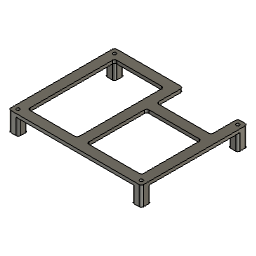
CCMDebugSupportv1 (Autodesk Fusion 360 design; units mm, degrees)
Autodesk Fusion 360 part; units mm, degrees
sketch "Sketch1" plane through (0, 0, 0) normal (0, 0, 1) x (1, 0, 0)
  line L0 (-60, 47.5) -> (60, 47.5)
  line L1 (60, 47.5) -> (60, -47.5)
  line L2 (60, -47.5) -> (-60, -47.5)
  line L3 (-60, -47.5) -> (-60, 47.5)
  line L4 (0, 66) -> (0, -78) construction
  line L5 (-80, 0) -> (100, 0) construction
  circle A0 centre (-57.5, 45) radius 1.5
  circle A1 centre (57.5, 45) radius 1.5
  circle A2 centre (-57.5, -45) radius 1.5
  circle A3 centre (57.5, -45) radius 1.5
  line L6 (62, -49.5) -> (-62, -49.5)
  line L7 (-62, -49.5) -> (-62, 49.5)
  line L8 (-62, 49.5) -> (62, 49.5)
  line L9 (62, 49.5) -> (62, -49.5)
  dimension "d1" = 120
  dimension "d2" = 95
  dimension "d3" = 3
  dimension "d4" = 2.5
  dimension "d5" = 2.5
  dimension "d8" = 115
  dimension "d9" = -90
  dimension "d12" = -2
  constraint horizontal L0
  constraint perpendicular L0 L1
  constraint parallel L0 L2
  constraint parallel L1 L3
  constraint perpendicular L2 L4
  constraint perpendicular L1 L5
  measures "d1" distance of L1.end L2.end
  measures "d2" distance of L0.end L1.end
  measures "d3" diameter of A0
  measures "d4" distance of L3 A0.centre
  measures "d5" distance of L0 A0.centre
extrude "Extrude1" add sketch "Sketch1" along normal blind 3 contours L0 L1 L2 L3
extrude "Extrude2" add sketch "Sketch1" along normal blind 3 contours L6 L7 L8 L9
sketch "Sketch2" plane through (0, 0, 3) normal (0, 0, 1) x (-1, 0, 0)
  line L0 (-62, -49.5) -> (62, -49.5)
  line L1 (62, -49.5) -> (62, 49.5)
  line L2 (62, 49.5) -> (-62, 49.5)
  line L3 (-62, 49.5) -> (-62, -49.5)
  circle A0 centre (57.5, -45) radius 1.5
  circle A1 centre (-57.5, -45) radius 1.5
  circle A2 centre (57.5, 45) radius 1.5
  circle A3 centre (-57.5, 45) radius 1.5
  line L4 (-2, -49.5) -> (-53, -49.5)
  line L5 (-53, -49.5) -> (-53, -24.5)
  line L6 (-53, -24.5) -> (-2, -24.5)
  line L7 (-2, -24.5) -> (-2, -49.5)
  dimension "d15" = 51
  dimension "d16" = 25
  dimension "d17" = 9
  constraint horizontal L4
  constraint vertical L5
  constraint horizontal L6
  constraint vertical L7
  constraint coincident L0 L4.start
  measures "d15" distance of L5.end L6.end
  measures "d16" distance of L4.start L6.end
  measures "d17" distance of L3 L5
extrude "Extrude3" cut sketch "Sketch2" against normal up to surface (3 mm away) contours L0 L4 L5 L6 L7
sketch "Sketch3" plane through (0, 0, 3) normal (0, 0, 1) x (-1, 0, 0)
  line L0 (-2, -24.5) -> (-2, -49.5)
  line L1 (-2, -49.5) -> (62, -49.5)
  line L2 (62, -49.5) -> (62, 49.5)
  line L3 (62, 49.5) -> (-62, 49.5)
  line L4 (-62, 49.5) -> (-62, -49.5)
  line L5 (-62, -49.5) -> (-53, -49.5)
  line L6 (-53, -49.5) -> (-53, -24.5)
  line L7 (-53, -24.5) -> (-2, -24.5)
  circle A0 centre (57.5, -45) radius 1.5
  circle A1 centre (-57.5, -45) radius 1.5
  circle A2 centre (57.5, 45) radius 1.5
  circle A3 centre (-57.5, 45) radius 1.5
  line L8 (53, -40.5) -> (7, -40.5)
  line L9 (7, -40.5) -> (7, 40.5)
  line L10 (7, 40.5) -> (53, 40.5)
  line L11 (53, 40.5) -> (53, -40.5)
  line L12 (-2, -15.5) -> (-53, -15.5)
  line L13 (-53, -15.5) -> (-53, 40.5)
  line L14 (-53, 40.5) -> (-2, 40.5)
  line L15 (-2, 40.5) -> (-2, -15.5)
  point P0 (57.5, -45)
  dimension "d20" = 4.5
  dimension "d21" = 4.5
  dimension "d22" = 4.5
  dimension "d23" = 4.5
  dimension "d24" = 9
  dimension "d25" = 4.5
  dimension "d27" = 9
  dimension "d28" = 9
  constraint horizontal L8
  constraint vertical L9
  constraint horizontal L10
  constraint vertical L11
  constraint horizontal L12
  constraint vertical L13
  constraint horizontal L14
  constraint vertical L15
  measures "d20" distance of P0 L8
  measures "d21" distance of L11 P0
  measures "d22" distance of A2.centre L10
  measures "d23" distance of A3.centre L13
  measures "d24" distance of L7 L12
  measures "d25" distance of A3.centre L14
  measures "d27" distance of L0 L9
  measures "d28" distance of L9 L15
extrude "Extrude4" cut sketch "Sketch3" against normal up to surface (3 mm away) contours L8 L9 L10 L11 | L12 L13 L14 L15
sketch "Sketch9" plane through (0, 0, 0) normal (0, 0, 1) x (1, 0, 0)
  line L0 (-62, -49.5) -> (-53, -49.5)
  line L1 (-53, -49.5) -> (-53, -40.5)
  line L2 (-53, -40.5) -> (-62, -40.5)
  line L3 (-62, -40.5) -> (-62, -49.5)
  line L4 (-62, -49.5) -> (-53, -40.5) construction
  line L5 (-53, -49.5) -> (-62, -40.5) construction
  line L6 (53, -49.5) -> (62, -49.5)
  line L7 (62, -49.5) -> (62, -40.5)
  line L8 (62, -40.5) -> (53, -40.5)
  line L9 (53, -40.5) -> (53, -49.5)
  line L10 (-62, 40.5) -> (-53, 40.5)
  line L11 (-53, 40.5) -> (-53, 49.5)
  line L12 (-53, 49.5) -> (-62, 49.5)
  line L13 (-62, 49.5) -> (-62, 40.5)
  line L14 (53, 40.5) -> (62, 40.5)
  line L15 (62, 40.5) -> (62, 49.5)
  line L16 (62, 49.5) -> (53, 49.5)
  line L17 (53, 49.5) -> (53, 40.5)
  point P0 (-57.5, -45)
  point P1 (-62, -49.5)
  point P2 (-57.5, -45)
  point P3 (57.5, -45)
  point P4 (-57.5, 45)
  point P5 (57.5, 45)
  dimension "d54" = 115
  dimension "d55" = 90
  constraint horizontal L0
  constraint perpendicular L0 L1
  constraint parallel L0 L2
  constraint parallel L1 L3
  constraint coincident L4 P2
  constraint coincident L5 P2
  constraint coincident L0.start L3.end
  constraint coincident P2 P0
extrude "Extrude10" add sketch "Sketch9" against normal blind 15
extrude "Extrude11" cut sketch "Sketch1" against normal up to surface (15 mm away) contours A0 | A1 | A2 | A3
fillet "Fillet1" radius 2 16 edges at (53, 49.5, -6) (2, 49.5, 1.5) (-53, 49.5, -7.5) (-62, 49.5, -6) (-62, -40.5, -7.5) (-53, -40.5, -7.5) (62, -40.5, -7.5) (53, -40.5, -7.5) (53, -49.5, -7.5) (-53, 40.5, -7.5) (53, 40.5, -7.5) (62, 40.5, -7.5) (-62, 40.5, -7.5) (-62, -49.5, -6) (62, -49.5, -6) (62, 49.5, -6)
fillet "Fillet2" radius 2 1 edges at (-53, -49.5, -7.5)
fillet "Fillet3" radius 2 10 edges at (53, 24.5, 1.5) (53, -40.5, 1.5) (53, 15.5, 1.5) (-7, 40.5, 1.5) (-7, -40.5, 1.5) (-53, -40.5, 1.5) (2, 24.5, 1.5) (-53, 40.5, 1.5) (2, -40.5, 1.5) (2, 15.5, 1.5)
equation "d20 = d22"
equation "d21 = d22"
equation "d23 = d22"
equation "d25 = d22"
equation "PillarHeight = 15 mm"
equation "d56 = -PillarHeight"
